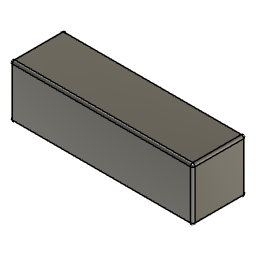
ripobattery (Autodesk Fusion 360 design; units mm, degrees)
Autodesk Fusion 360 part; units mm, degrees
sketch "スケッチ1" plane through (0, 0, 0) normal (0, 0, 1) x (1, 0, 0)
  line L0 (0, 0) -> (115.8, 0)
  line L1 (115.8, 0) -> (115.8, 33.8)
  line L2 (115.8, 33.8) -> (0, 33.8)
  line L3 (0, 33.8) -> (0, 0)
  dimension "d1" = 115.8
  dimension "d2" = 33.8
  constraint horizontal L0
  constraint vertical L1
  constraint horizontal L2
  constraint vertical L3
  constraint coincident L0.start L3.end
  measures "d1" distance of L0.start L0.end
  measures "d2" distance of L0.start L2.end
extrude "押し出し1" add sketch "スケッチ1" along normal blind 33.8
fillet "フィレット1" radius 1.5 4 faces at (38.6, 22.5333, 33.8) (38.6, 22.5333, 0) (38.6, 0, 11.2667) (77.2, 33.8, 11.2667)
